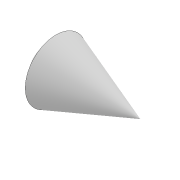
# Autodesk Inventor part: 錐
Saved by Autodesk Inventor 2022 (Build 260153000, 153)
## iProperties
Created: 2023-10-13
Part Number: 錐
Material: 一般
Document SubType Name: Modeling
Designer: JOU
Density: 1 g/cm^3
Appearance: 預設
Author: JOU
Autodesk Inventor part; units mm, degrees
ref_plane "YZ Plane" through (0, 0, 0) normal (1, 0, 0) x (0, 1, 0)
ref_plane "XZ Plane" through (0, 0, 0) normal (0, 1, 0) x (-1, 0, 0)
ref_plane "XY Plane" through (0, 0, 0) normal (0, 0, 1) x (1, 0, 0)
sketch "草圖1" plane through (0, 0, 0) normal (0, 0, 1) x (1, 0, 0)
  spline S0 degree 3 poles (33.0704, -1.028) (33.1128, -1.3407) (33.229, -1.9203) (33.4717, -2.7083) (33.728, -3.3729) (33.974, -3.9444) (34.2027, -4.4575) (34.4141, -4.9414) (34.6098, -5.4181) (34.79, -5.903) (34.9532, -6.4067) (35.0962, -6.9355) (35.2148, -7.4925) (35.3042, -8.0783) (35.3596, -8.6912) (35.3762, -9.3277) (35.3502, -9.9827) (35.2785, -10.6504) (35.1591, -11.3236) (34.9915, -11.9952) (34.7762, -12.6575) (34.5154, -13.3032) (34.2121, -13.9254) (33.8708, -14.5179) (33.4966, -15.0755) (33.0955, -15.594) (32.6736, -16.0709) (32.2373, -16.5048) (31.7922, -16.896) (31.3433, -17.2465) (30.8938, -17.5596) (30.4451, -17.8406) (29.9953, -18.0963) (29.5391, -18.3356) (29.066, -18.5704) (28.561, -18.8165) (28.0052, -19.0962) (27.3817, -19.4405) (26.6891, -19.8881) (25.9593, -20.4728) (25.2612, -21.1967) (24.6696, -22.0099) (24.2205, -22.8301) (23.8999, -23.5899) (23.6691, -24.2637) (23.4902, -24.8597) (23.3355, -25.3997) (23.1865, -25.9063) (23.03, -26.3973) (22.8563, -26.8846) (22.6575, -27.3753) (22.4272, -27.8723) (22.16, -28.3752) (21.852, -28.8815) (21.5004, -29.3866) (21.1041, -29.8848) (20.663, -30.3699) (20.1789, -30.8352) (19.6547, -31.2743) (19.0947, -31.6809) (18.5041, -32.05) (17.8892, -32.3769) (17.2569, -32.6586) (16.6146, -32.8931) (15.9696, -33.0797) (15.329, -33.2191) (14.6993, -33.3132) (14.0861, -33.3651) (13.4937, -33.3787) (12.9245, -33.3586) (12.3789, -33.3096) (11.8546, -33.2364) (11.3457, -33.1432) (10.8423, -33.0332) (10.329, -32.909) (9.784, -32.7729) (9.1784, -32.6299) (8.4795, -32.4929) (7.6612, -32.3906) (6.7263, -32.3694) (5.7263, -32.4752) (4.7503, -32.7179) (3.8791, -33.0575) (3.1451, -33.4335) (2.5352, -33.8013) (2.015, -34.1428) (1.5494, -34.4571) (1.1096, -34.7494) (0.6742, -35.0249) (0.2279, -35.2865) (-0.2398, -35.5347) (-0.7357, -35.7673) (-1.2637, -35.9809) (-1.8251, -36.1707) (-2.419, -36.3316) (-3.0429, -36.4585) (-3.6926, -36.5466) (-4.3625, -36.5919) (-5.0463, -36.5913) (-5.7368, -36.5428) (-6.4264, -36.4459) (-7.1076, -36.3011) (-7.773, -36.1105) (-8.4157, -35.8772) (-9.0298, -35.6056) (-9.6101, -35.3006) (-10.153, -34.9679) (-10.6561, -34.6135) (-11.1187, -34.2432) (-11.5418, -33.8619) (-11.9282, -33.4737) (-12.2828, -33.0806) (-12.6127, -32.682) (-12.9277, -32.2742) (-13.241, -31.8492) (-13.571, -31.3946) (-13.943, -30.8957) (-14.3904, -30.3415) (-14.9515, -29.7372) (-15.654, -29.12) (-16.4881, -28.5582) (-17.3917, -28.1168) (-18.2774, -27.8169) (-19.0813, -27.6332) (-19.785, -27.5229) (-20.403, -27.4502) (-20.9617, -27.3916) (-21.4865, -27.3328) (-21.9971, -27.264) (-22.5072, -27.1775) (-23.0249, -27.067) (-23.5544, -26.9264) (-24.0961, -26.7506) (-24.6482, -26.5352) (-25.2066, -26.2767) (-25.7661, -25.9729) (-26.3204, -25.6228) (-26.8627, -25.2269) (-27.3861, -24.7869) (-27.8839, -24.3059) (-28.3499, -23.7884) (-28.7786, -23.2396) (-29.1658, -22.6659) (-29.5083, -22.074) (-29.804, -21.4712) (-30.0525, -20.8645) (-30.2546, -20.2607) (-30.4122, -19.6659) (-30.5285, -19.0848) (-30.6075, -18.5208) (-30.654, -17.975) (-30.673, -17.4459) (-30.6695, -16.9286) (-30.6487, -16.4138) (-30.6155, -15.8867) (-30.5761, -15.3264) (-30.5404, -14.7051) (-30.5268, -13.993) (-30.5682, -13.1694) (-30.7097, -12.245) (-30.9875, -11.2785) (-31.3959, -10.3595) (-31.8817, -9.5605) (-32.3794, -8.903) (-32.8475, -8.3662) (-33.2742, -7.9133) (-33.6646, -7.5093) (-34.0288, -7.1269) (-34.3757, -6.7459) (-34.7109, -6.3519) (-35.0364, -5.9344) (-35.3517, -5.4864) (-35.6537, -5.0035) (-35.9381, -4.4836) (-36.1997, -3.9266) (-36.433, -3.3343) (-36.6326, -2.7098) (-36.7936, -2.0579) (-36.9117, -1.3844) (-36.9838, -0.696) (-37.0081, 0) (-36.9838, 0.696) (-36.9117, 1.3844) (-36.7936, 2.0579) (-36.6326, 2.7098) (-36.433, 3.3343) (-36.1997, 3.9266) (-35.9381, 4.4836) (-35.6537, 5.0035) (-35.3517, 5.4864) (-35.0364, 5.9344) (-34.7109, 6.3519) (-34.3757, 6.7459) (-34.0288, 7.1269) (-33.6646, 7.5093) (-33.2742, 7.9133) (-32.8475, 8.3662) (-32.3794, 8.903) (-31.8817, 9.5605) (-31.3959, 10.3595) (-30.9875, 11.2785) (-30.7097, 12.245) (-30.5682, 13.1694) (-30.5268, 13.993) (-30.5404, 14.7051) (-30.5761, 15.3264) (-30.6155, 15.8867) (-30.6487, 16.4138) (-30.6695, 16.9286) (-30.673, 17.4459) (-30.654, 17.975) (-30.6075, 18.5208) (-30.5285, 19.0848) (-30.4122, 19.6659) (-30.2546, 20.2607) (-30.0525, 20.8645) (-29.804, 21.4712) (-29.5083, 22.074) (-29.1658, 22.6659) (-28.7786, 23.2396) (-28.3499, 23.7884) (-27.8839, 24.3059) (-27.3861, 24.7869) (-26.8627, 25.2269) (-26.3204, 25.6228) (-25.7661, 25.9729) (-25.2066, 26.2767) (-24.6482, 26.5352) (-24.0961, 26.7506) (-23.5544, 26.9264) (-23.0249, 27.067) (-22.5072, 27.1775) (-21.9971, 27.264) (-21.4865, 27.3328) (-20.9617, 27.3916) (-20.403, 27.4502) (-19.785, 27.5229) (-19.0813, 27.6332) (-18.2774, 27.8169) (-17.3917, 28.1168) (-16.4881, 28.5582) (-15.654, 29.12) (-14.9515, 29.7372) (-14.3904, 30.3415) (-13.943, 30.8957) (-13.571, 31.3946) (-13.241, 31.8492) (-12.9277, 32.2742) (-12.6127, 32.682) (-12.2828, 33.0806) (-11.9282, 33.4737) (-11.5418, 33.8619) (-11.1187, 34.2432) (-10.6561, 34.6135) (-10.153, 34.9679) (-9.6101, 35.3006) (-9.0298, 35.6056) (-8.4157, 35.8772) (-7.773, 36.1105) (-7.1076, 36.3011) (-6.4264, 36.4459) (-5.7368, 36.5428) (-5.0463, 36.5913) (-4.3625, 36.5919) (-3.6926, 36.5466) (-3.0429, 36.4585) (-2.419, 36.3316) (-1.8251, 36.1707) (-1.2637, 35.9809) (-0.7357, 35.7673) (-0.2398, 35.5347) (0.2279, 35.2865) (0.6742, 35.0249) (1.1096, 34.7494) (1.5494, 34.4571) (2.015, 34.1428) (2.5352, 33.8013) (3.1451, 33.4335) (3.8791, 33.0575) (4.7503, 32.7179) (5.7263, 32.4752) (6.7263, 32.3694) (7.6612, 32.3906) (8.4795, 32.4929) (9.1784, 32.6299) (9.784, 32.7729) (10.329, 32.909) (10.8423, 33.0332) (11.3457, 33.1432) (11.8546, 33.2364) (12.3789, 33.3096) (12.9245, 33.3586) (13.4937, 33.3787) (14.0861, 33.3651) (14.6993, 33.3132) (15.329, 33.2191) (15.9696, 33.0797) (16.6146, 32.8931) (17.2569, 32.6586) (17.8892, 32.3769) (18.5041, 32.05) (19.0947, 31.6809) (19.6547, 31.2743) (20.1789, 30.8352) (20.663, 30.3699) (21.1041, 29.8848) (21.5004, 29.3866) (21.852, 28.8815) (22.16, 28.3752) (22.4272, 27.8723) (22.6575, 27.3753) (22.8563, 26.8846) (23.03, 26.3973) (23.1865, 25.9063) (23.3355, 25.3997) (23.4902, 24.8597) (23.6691, 24.2637) (23.8999, 23.5899) (24.2205, 22.8301) (24.6696, 22.0099) (25.2612, 21.1967) (25.9593, 20.4728) (26.6891, 19.8881) (27.3817, 19.4405) (28.0052, 19.0962) (28.561, 18.8165) (29.066, 18.5704) (29.5391, 18.3356) (29.9953, 18.0963) (30.4451, 17.8406) (30.8938, 17.5596) (31.3433, 17.2465) (31.7922, 16.896) (32.2373, 16.5048) (32.6736, 16.0709) (33.0955, 15.594) (33.4966, 15.0755) (33.8708, 14.5179) (34.2121, 13.9254) (34.5154, 13.3032) (34.7762, 12.6575) (34.9915, 11.9952) (35.1591, 11.3236) (35.2785, 10.6504) (35.3502, 9.9827) (35.3762, 9.3277) (35.3596, 8.6912) (35.3042, 8.0783) (35.2148, 7.4925) (35.0962, 6.9355) (34.9532, 6.4067) (34.79, 5.903) (34.6098, 5.4181) (34.4141, 4.9414) (34.2027, 4.4575) (33.974, 3.9444) (33.728, 3.3729) (33.4717, 2.7083) (33.2289, 1.9202) (33.0457, 1.0032) (32.976, 0.0001) (33.0242, -0.6877) (33.0704, -1.028) knots 0 0 0 0 0.004014 0.007499 0.010478 0.013071 0.015414 0.017624 0.019788 0.021968 0.024203 0.026521 0.028933 0.031445 0.034054 0.036756 0.039538 0.042388 0.045291 0.048229 0.051186 0.054143 0.057081 0.059984 0.062834 0.065617 0.068318 0.070928 0.07344 0.075852 0.078169 0.080405 0.082584 0.084748 0.086958 0.089302 0.091894 0.094873 0.098359 0.102372 0.106742 0.111111 0.115125 0.11861 0.121589 0.124182 0.126525 0.128735 0.130899 0.133079 0.135315 0.137632 0.140044 0.142556 0.145166 0.147867 0.150649 0.153499 0.156402 0.159341 0.162297 0.165254 0.168192 0.171095 0.173945 0.176728 0.179429 0.182039 0.184551 0.186963 0.18928 0.191516 0.193695 0.195859 0.198069 0.200413 0.203006 0.205984 0.20947 0.213483 0.217853 0.222222 0.226236 0.229721 0.2327 0.235293 0.237636 0.239846 0.24201 0.24419 0.246426 0.248743 0.251155 0.253667 0.256277 0.258978 0.26176 0.26461 0.267513 0.270452 0.273408 0.276365 0.279304 0.282206 0.285056 0.287839 0.29054 0.29315 0.295662 0.298074 0.300391 0.302627 0.304806 0.306971 0.309181 0.311524 0.314117 0.317096 0.320581 0.324594 0.328964 0.333333 0.337347 0.340832 0.343811 0.346404 0.348747 0.350957 0.353121 0.355301 0.357537 0.359854 0.362266 0.364778 0.367388 0.370089 0.372871 0.375722 0.378624 0.381563 0.384519 0.387476 0.390415 0.393317 0.396168 0.39895 0.401651 0.404261 0.406773 0.409185 0.411502 0.413738 0.415918 0.418082 0.420292 0.422635 0.425228 0.428207 0.431692 0.435706 0.440075 0.444444 0.448458 0.451943 0.454922 0.457515 0.459858 0.462068 0.464232 0.466412 0.468648 0.470965 0.473377 0.475889 0.478499 0.4812 0.483982 0.486833 0.489735 0.492674 0.495631 0.498587 0.501526 0.504428 0.507279 0.510061 0.512762 0.515372 0.517884 0.520296 0.522613 0.524849 0.527029 0.529193 0.531403 0.533746 0.536339 0.539318 0.542803 0.546817 0.551186 0.555556 0.559569 0.563054 0.566033 0.568626 0.570969 0.573179 0.575344 0.577523 0.579759 0.582076 0.584488 0.587 0.58961 0.592311 0.595094 0.597944 0.600846 0.603785 0.606742 0.609698 0.612637 0.61554 0.61839 0.621172 0.623873 0.626483 0.628995 0.631407 0.633724 0.63596 0.63814 0.640304 0.642514 0.644857 0.64745 0.650429 0.653914 0.657928 0.662297 0.666667 0.67068 0.674166 0.677144 0.679737 0.682081 0.684291 0.686455 0.688634 0.69087 0.693187 0.695599 0.698111 0.700721 0.703422 0.706205 0.709055 0.711958 0.714896 0.717853 0.720809 0.723748 0.726651 0.729501 0.732283 0.734984 0.737594 0.740106 0.742518 0.744835 0.747071 0.749251 0.751415 0.753625 0.755968 0.758561 0.76154 0.765025 0.769039 0.773408 0.777778 0.781791 0.785277 0.788256 0.790848 0.793192 0.795402 0.797566 0.799745 0.801981 0.804298 0.80671 0.809222 0.811832 0.814533 0.817316 0.820166 0.823069 0.826007 0.828964 0.831921 0.834859 0.837762 0.840612 0.843394 0.846096 0.848705 0.851217 0.853629 0.855947 0.858182 0.860362 0.862526 0.864736 0.867079 0.869672 0.872651 0.876136 0.88015 0.884519 0.888889 0.892902 0.896388 0.899367 0.901959 0.904303 0.906513 0.908677 0.910856 0.913092 0.915409 0.917822 0.920333 0.922943 0.925645 0.928427 0.931277 0.93418 0.937118 0.940075 0.943032 0.94597 0.948873 0.951723 0.954505 0.957207 0.959817 0.962328 0.964741 0.967058 0.969294 0.971473 0.973637 0.975847 0.978191 0.980783 0.983762 0.987248 0.991261 0.995631 1 1 1 1
  line L0 (0, 0) -> (-31.0099, 11.2867)
  line L1 (0, 0) -> (-31.0099, -11.2867)
  line L2 (0, 0) -> (-37, 0)
  point P0 (33.4931, -2.7429)
  point P1 (33.7434, -3.3994)
  point P2 (33.983, -3.9619)
  point P3 (34.2063, -4.4674)
  point P4 (34.4138, -4.9455)
  point P5 (34.6067, -5.418)
  point P6 (34.7851, -5.9001)
  point P7 (34.9471, -6.4018)
  point P8 (35.0895, -6.9294)
  point P9 (35.2078, -7.4858)
  point P10 (35.2972, -8.0714)
  point P11 (35.3525, -8.6844)
  point P12 (35.3692, -9.3212)
  point P13 (35.3432, -9.9769)
  point P14 (35.2714, -10.6452)
  point P15 (35.1519, -11.3192)
  point P16 (34.9841, -11.9916)
  point P17 (34.7686, -12.6547)
  point P18 (34.5074, -13.3013)
  point P19 (34.2038, -13.9242)
  point P20 (33.862, -14.5173)
  point P21 (33.4874, -15.0754)
  point P22 (33.0859, -15.5944)
  point P23 (32.6638, -16.0715)
  point P24 (32.2274, -16.5055)
  point P25 (31.7826, -16.8967)
  point P26 (31.3343, -17.2469)
  point P27 (30.8861, -17.5595)
  point P28 (30.4394, -17.8397)
  point P29 (29.9929, -18.0943)
  point P30 (29.5414, -18.3323)
  point P31 (29.0751, -18.5652)
  point P32 (28.5792, -18.8089)
  point P33 (28.034, -19.0858)
  point P34 (27.4203, -19.4277)
  point P35 (26.7315, -19.8762)
  point P36 (25.9942, -20.4697)
  point P37 (25.2795, -21.212)
  point P38 (24.6726, -22.0447)
  point P39 (24.2161, -22.8739)
  point P40 (23.894, -23.6301)
  point P41 (23.6638, -24.2939)
  point P42 (23.4859, -24.8788)
  point P43 (23.332, -25.4096)
  point P44 (23.1836, -25.9092)
  point P45 (23.0276, -26.3952)
  point P46 (22.8544, -26.8791)
  point P47 (22.656, -27.3677)
  point P48 (22.426, -27.8633)
  point P49 (22.159, -28.3656)
  point P50 (21.851, -28.8716)
  point P51 (21.4994, -29.3768)
  point P52 (21.1028, -29.8754)
  point P53 (20.6614, -30.3609)
  point P54 (20.1769, -30.8267)
  point P55 (19.6521, -31.2663)
  point P56 (19.0913, -31.6735)
  point P57 (18.5, -32.0429)
  point P58 (17.8844, -32.3703)
  point P59 (17.2513, -32.6523)
  point P60 (16.6083, -32.887)
  point P61 (15.9626, -33.0738)
  point P62 (15.3214, -33.2132)
  point P63 (14.6914, -33.3074)
  point P64 (14.0781, -33.3593)
  point P65 (13.4859, -33.373)
  point P66 (12.9174, -33.3531)
  point P67 (12.3731, -33.3045)
  point P68 (11.8508, -33.2321)
  point P69 (11.3451, -33.1401)
  point P70 (10.8463, -33.0322)
  point P71 (10.3394, -32.9109)
  point P72 (9.8028, -32.7788)
  point P73 (9.2072, -32.6404)
  point P74 (8.5173, -32.5079)
  point P75 (7.7014, -32.4087)
  point P76 (6.755, -32.3894)
  point P77 (5.7304, -32.4987)
  point P78 (4.7302, -32.7465)
  point P79 (3.8475, -33.0882)
  point P80 (3.1147, -33.4605)
  point P81 (2.5118, -33.821)
  point P82 (1.9994, -34.1547)
  point P83 (1.5404, -34.4624)
  point P84 (1.1055, -34.7497)
  point P85 (0.6737, -35.0218)
  point P86 (0.2299, -35.2812)
  point P87 (-0.2361, -35.5279)
  point P88 (-0.7309, -35.7597)
  point P89 (-1.2583, -35.9728)
  point P90 (-1.8195, -36.1625)
  point P91 (-2.4136, -36.3235)
  point P92 (-3.0378, -36.4505)
  point P93 (-3.688, -36.5387)
  point P94 (-4.3587, -36.5841)
  point P95 (-5.0432, -36.5835)
  point P96 (-5.7345, -36.5349)
  point P97 (-6.425, -36.4379)
  point P98 (-7.107, -36.2929)
  point P99 (-7.7732, -36.1021)
  point P100 (-8.4167, -35.8685)
  point P101 (-9.0313, -35.5965)
  point P102 (-9.6122, -35.2912)
  point P103 (-10.1553, -34.9584)
  point P104 (-10.6585, -34.604)
  point P105 (-11.121, -34.2338)
  point P106 (-11.5437, -33.8531)
  point P107 (-11.9294, -33.466)
  point P108 (-12.2829, -33.0748)
  point P109 (-12.6112, -32.6793)
  point P110 (-12.924, -32.276)
  point P111 (-13.2343, -31.8572)
  point P112 (-13.5604, -31.4111)
  point P113 (-13.9277, -30.9223)
  point P114 (-14.3711, -30.3773)
  point P115 (-14.9323, -29.7768)
  point P116 (-15.6449, -29.1538)
  point P117 (-16.5, -28.5788)
  point P118 (-17.4255, -28.1258)
  point P119 (-18.3213, -27.8202)
  point P120 (-19.122, -27.6344)
  point P121 (-19.8156, -27.5229)
  point P122 (-20.4226, -27.4492)
  point P123 (-20.972, -27.3899)
  point P124 (-21.4898, -27.3305)
  point P125 (-21.9955, -27.2613)
  point P126 (-22.5022, -27.1747)
  point P127 (-23.0177, -27.0642)
  point P128 (-23.5458, -26.9237)
  point P129 (-24.0868, -26.748)
  point P130 (-24.6386, -26.5325)
  point P131 (-25.1972, -26.274)
  point P132 (-25.757, -25.97)
  point P133 (-26.3118, -25.6196)
  point P134 (-26.8547, -25.2233)
  point P135 (-27.3787, -24.7828)
  point P136 (-27.8771, -24.3013)
  point P137 (-28.3436, -23.7831)
  point P138 (-28.7729, -23.2337)
  point P139 (-29.1606, -22.6593)
  point P140 (-29.5034, -22.0667)
  point P141 (-29.7994, -21.4633)
  point P142 (-30.0481, -20.8561)
  point P143 (-30.2503, -20.252)
  point P144 (-30.4079, -19.657)
  point P145 (-30.5242, -19.0762)
  point P146 (-30.6033, -18.5128)
  point P147 (-30.65, -17.9684)
  point P148 (-30.6693, -17.4415)
  point P149 (-30.6666, -16.9274)
  point P150 (-30.6469, -16.4175)
  point P151 (-30.6155, -15.8972)
  point P152 (-30.5786, -15.3458)
  point P153 (-30.5457, -14.7353)
  point P154 (-30.535, -14.0328)
  point P155 (-30.579, -13.2121)
  point P156 (-30.7244, -12.2768)
  point P157 (-31.4276, -10.3447)
  point P158 (-31.9174, -9.5348)
  point P159 (-32.4113, -8.8778)
  point P160 (-32.871, -8.3466)
  point P161 (-33.2886, -7.8999)
  point P162 (-33.6714, -7.5013)
  point P163 (-34.0298, -7.1229)
  point P164 (-34.3727, -6.7449)
  point P165 (-34.7052, -6.3529)
  point P166 (-35.0291, -5.9369)
  point P167 (-35.3433, -5.4898)
  point P168 (-35.6448, -5.0074)
  point P169 (-35.9291, -4.4877)
  point P170 (-36.1907, -3.9306)
  point P171 (-36.4242, -3.3379)
  point P172 (-36.624, -2.7129)
  point P173 (-36.7851, -2.0603)
  point P174 (-36.9034, -1.3861)
  point P175 (-36.9757, -0.6968)
  point P176 (-36.9757, 0.6968)
  point P177 (-36.9034, 1.3861)
  point P178 (-36.7851, 2.0603)
  point P179 (-36.624, 2.7129)
  point P180 (-36.4242, 3.3379)
  point P181 (-36.1907, 3.9306)
  point P182 (-35.9291, 4.4877)
  point P183 (-35.6448, 5.0074)
  point P184 (-35.3433, 5.4898)
  point P185 (-35.0291, 5.9369)
  point P186 (-34.7052, 6.3529)
  point P187 (-34.3727, 6.7449)
  point P188 (-34.0298, 7.1229)
  point P189 (-33.6714, 7.5013)
  point P190 (-33.2886, 7.8999)
  point P191 (-32.871, 8.3466)
  point P192 (-32.4113, 8.8778)
  point P193 (-31.9174, 9.5348)
  point P194 (-31.4276, 10.3447)
  point P195 (-30.7244, 12.2768)
  point P196 (-30.579, 13.2121)
  point P197 (-30.535, 14.0328)
  point P198 (-30.5457, 14.7353)
  point P199 (-30.5786, 15.3458)
  constraints: 6 end point, 1 horizontal, 360 other
revolve "迴轉2" add sketch "草圖1" angle 360 about axis through (0, 0, 0) along (-1, 0, 0) contours L0 L2 S0
